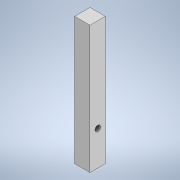
# Autodesk Inventor part: lever
Saved by Autodesk Inventor 2020.2 (Build 242310000, 310)
## iProperties
Created: 2020-02-28
Part Number: lever
Material: Generic
Document SubType Name: Modeling
Designer: ColinP
Density: 1 g/cm^3
Appearance: Default
Author: ColinP
Autodesk Inventor part; units mm, degrees
ref_plane "YZ Plane" through (0, 0, 0) normal (1, 0, 0) x (0, 1, 0)
ref_plane "XZ Plane" through (0, 0, 0) normal (0, 1, 0) x (-1, 0, 0)
ref_plane "XY Plane" through (0, 0, 0) normal (0, 0, 1) x (1, 0, 0)
sketch "Sketch1" plane through (0, 0, 0) normal (0, 0, 1) x (1, 0, 0)
  line L0 (-8.0472, 18.8479) -> (1.9528, 18.8479)
  line L1 (1.9528, 18.8479) -> (1.9528, -64.3521)
  line L2 (1.9528, -64.3521) -> (-8.0472, -64.3521)
  line L3 (-8.0472, -64.3521) -> (-8.0472, 18.8479)
  point P0 (0, 0)
  dimension "d0" = 10
  dimension "d1" = 83.2
  constraints: 8 end point, 2 parallel, 1 horizontal, 1 perpendicular
  measures "d0" distance of L1.end L2.end
  measures "d1" distance of L0.end L1.end
extrude "Extrusion1" add sketch "Sketch1" along normal blind 10
sketch "Sketch2" plane through (1.9528, -64.3521, 0) normal (1, 0, 0) x (0, 0, -1)
  line L0 (0, 83.2) -> (-10, 83.2) projected
  line L1 (-5, 83.2) -> (-5, 22.4)
  point P0 (0, 64.3521)
  dimension "d4" = 60.8
  constraints: 2 end point, 1 midpoint, 1 vertical
  measures "d4" distance of L1.start L1.end
hole "Hole1" at (1.9528, -41.9521, 5) direction (-1, 0, 0) diameter 3.6 end through all clearance for "Flat Head Machine Screw" size "M3" standard "Ansi Metric M Profile"
body "Solid1"
